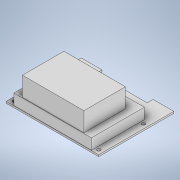
# Autodesk Inventor part: JetsonXavierNX_and_EN715
Saved by Autodesk Inventor 2020.4 (Build 244396000, 396)
## iProperties
Created: 2022-04-16
Part Number: JetsonXavierNX_and_EN715
Material: 一般
Document SubType Name: Modeling
Designer: Masato Kubotera
Density: 1 g/cm^3
Appearance: 既定
Author: Masato Kubotera
Autodesk Inventor part; units mm, degrees
ref_plane "YZ Plane" through (0, 0, 0) normal (1, 0, 0) x (0, 1, 0)
ref_plane "XZ Plane" through (0, 0, 0) normal (0, 1, 0) x (-1, 0, 0)
ref_plane "XY Plane" through (0, 0, 0) normal (0, 0, 1) x (1, 0, 0)
sketch "スケッチ1" plane through (0, 0, 0) normal (0, 0, 1) x (1, 0, 0)
  line L0 (35.3, 43.5) -> (-35.3, 43.5)
  line L1 (-35.3, 43.5) -> (-35.3, -43.5)
  line L2 (-35.3, -43.5) -> (35.3, -43.5)
  line L3 (35.3, 43.5) -> (-35.3, -43.5) construction
  line L4 (-35.3, 43.5) -> (35.3, -43.5) construction
  circle A0 centre (-31.3, -39.5) radius 1.6
  circle A1 centre (10.7, -39.5) radius 1.6
  line L5 (29.7, 0) -> (-35.3, 0) construction
  circle A2 centre (-31.3, 39.5) radius 1.6
  circle A3 centre (10.7, 39.5) radius 1.6
  line L6 (14.65, 36.45) -> (-35.1, 36.45)
  line L7 (-35.1, 36.45) -> (-35.1, -36.45)
  line L8 (-35.1, -36.45) -> (14.65, -36.45)
  line L9 (14.65, -36.45) -> (14.65, 36.45)
  line L10 (14.65, 36.45) -> (-35.1, -36.45) construction
  line L11 (-35.1, 36.45) -> (14.65, -36.45) construction
  line L12 (35.3, -24) -> (29.7, -24)
  line L13 (29.7, -24) -> (29.7, 24)
  line L14 (29.7, 24) -> (35.3, 24)
  line L15 (35.3, -43.5) -> (35.3, -24)
  line L16 (35.3, 24) -> (35.3, 43.5)
  line L17 (4.4, 28.9) -> (-34.6, 28.9)
  line L18 (-34.6, 28.9) -> (-34.6, -28.9)
  line L19 (-34.6, -28.9) -> (4.4, -28.9)
  line L20 (4.4, -28.9) -> (4.4, 28.9)
  line L21 (4.4, 28.9) -> (-34.6, -28.9) construction
  line L22 (-34.6, 28.9) -> (4.4, -28.9) construction
  point P0 (0, 0)
  point P1 (-10.225, 0)
  point P2 (-10.225, 0)
  point P3 (-15.1, 0)
  dimension "d0" = 70.6
  dimension "d1" = 87
  dimension "d2" = 3.2
  dimension "d3" = 3.2
  dimension "d4" = 4
  dimension "d5" = 46
  dimension "d6" = 4
  dimension "d7" = 4
  dimension "d8" = 49.75
  dimension "d9" = 72.9
  dimension "d10" = 0.2
  dimension "d11" = 19.5
  dimension "d12" = 5.6
  dimension "d13" = 39
  dimension "d14" = 57.8
  dimension "d15" = 7.55
  dimension "d16" = 0.5
  constraints: 46 end point, 9 midpoint, 7 parallel, 6 perpendicular, 4 centre point, 4 horizontal, 2 point on line, 2 symmetric about line, 1 collinear, 3 other
  measures "d0" distance of L2.end L1.end
  measures "d1" distance of L1.end L0.end
  measures "d2" diameter of A0
  measures "d3" diameter of A1
  measures "d4" distance from line of A0.centre L1
  measures "d5" distance from line of L1 A1.centre
  measures "d6" distance from line of L2 A0.centre
  measures "d7" distance from line of L2 A1.centre
  measures "d8" distance of L8.end L7.end
  measures "d9" distance of L7.end L6.end
  measures "d10" distance between parallel lines of L1 L7
  measures "d11" distance between parallel lines of L2 L12
  measures "d12" distance of L12.start L12.end
  measures "d13" distance of L19.end L18.end
  measures "d14" distance of L18.end L17.end
  measures "d15" distance between parallel lines of L8 L19
  measures "d16" distance between parallel lines of L18 L7
extrude "押し出し1" add sketch "スケッチ1" along normal blind 1.6 contours L16 L14 L13 L12 L15 L2 L1 L0 | L9 L8 L7 L6 | L20 L19 L18 L17
extrude "押し出し2" add sketch "スケッチ1" along normal blind 11.79 contours L9 L8 L7 L6 | L20 L19 L18 L17
extrude "押し出し3" add sketch "スケッチ1" along normal blind 29.79 contours L20 L19 L18 L17
equation "\"d7\" = d6"
